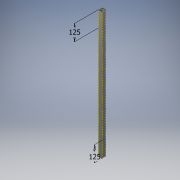
# Autodesk Inventor part: 1250mm_box_section
Saved by Autodesk Inventor 2019 (Build 230136000, 136)
## iProperties
Created: 2019-04-24
Part Number: 1250mm_box_section
Material: Steel, Mild
Document SubType Name: Modeling
Designer: callum.snowden
Density: 7.85 g/cm^3
Appearance: Semi-Polished
Mass: 2698.44 g
Surface Area: 2755.5 cm^2
Volume: 343.75 cm^3
Author: callum.snowden
Autodesk Inventor part; units mm, degrees
ref_plane "YZ Plane" through (0, 0, 0) normal (1, 0, 0) x (0, 1, 0)
ref_plane "XZ Plane" through (0, 0, 0) normal (0, 1, 0) x (-1, 0, 0)
ref_plane "XY Plane" through (0, 0, 0) normal (0, 0, 1) x (1, 0, 0)
sketch "Sketch1" plane through (0, 0, 0) normal (0, 1, 0) x (-1, 0, 0)
  line L0 (0, 0) -> (30, 0)
  line L1 (30, 0) -> (30, -30)
  line L2 (30, -30) -> (0, -30)
  line L3 (0, -30) -> (0, 0)
  line L4 (30, -15) -> (0, -15) construction
  line L5 (15, -30) -> (15, 0) construction
  line L6 (27.5, -2.5) -> (2.5, -2.5)
  line L7 (2.5, -2.5) -> (2.5, -27.5)
  line L8 (2.5, -27.5) -> (27.5, -27.5)
  line L9 (27.5, -27.5) -> (27.5, -2.5)
  dimension "d0" = 30
  dimension "d1" = 30
  dimension "d2" = 2.5
  dimension "d3" = 2.5
  constraints: 20 end point, 4 midpoint, 4 parallel, 2 horizontal, 2 perpendicular, 2 other
  measures "d0" distance of L1.end L2.end
  measures "d1" distance of L0.end L1.end
  measures "d2" distance between parallel lines of L0 L6
  measures "d3" distance between parallel lines of L1 L9
extrude "Extrusion1" add sketch "Sketch1" along normal blind 1000
sketch "Sketch2" plane through (0, 0, 0) normal (1, 0, 0) x (0, 0, -1)
  line L0 (30, 0) -> (0, 0) construction
  line L1 (30, 0) -> (30, 1000) construction
  line L2 (0, 1000) -> (30, 1000) construction
  line L3 (0, 0) -> (0, 1000) construction
  line L4 (0, 0) -> (0, 1000) construction
  line L5 (0, 125) -> (30, 125) construction
  line L6 (30, 0) -> (30, 1000) construction
  dimension "d6" = 125
  constraints: 2 end point, 2 point on line, 1 perpendicular
  measures "d6" distance between parallel lines of L0 L5
sketch "Sketch3" plane through (-30, 0, -30) normal (-1, 0, 0) x (0, 0, 1)
  line L0 (30, 0) -> (0, 0) construction
  line L1 (30, 0) -> (30, 1000) construction
  line L2 (0, 1000) -> (30, 1000) construction
  line L3 (0, 0) -> (0, 1000) construction
  line L4 (30, 125) -> (0, 125) construction
  line L5 (30, 0) -> (30, 1000) construction
  line L6 (30, 875) -> (1.3146, 875) construction
  line L7 (0, 0) -> (0, 1000) construction
  dimension "d7" = 125
  constraints: 2 end point, 1 perpendicular, 1 point on line
  measures "d7" distance between parallel lines of L2 L6
equation "\"d0\" = d1"
equation "\"d3\" = d2"
body "Solid1"
